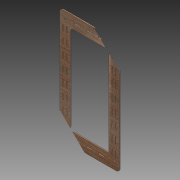
# Autodesk Inventor part: prim
Saved by Autodesk Inventor 2015 (Build 190159000, 159)
## iProperties
Created: 2015-12-31
Part Number: prim
Material: Generic
Document SubType Name: Modeling
Designer: david
Density: 1 g/cm^3
Appearance: Birch - Natural Polished
Author: david
Autodesk Inventor part; units mm, degrees
ref_plane "YZ Plane" through (0, 0, 0) normal (1, 0, 0) x (0, 1, 0)
ref_plane "XZ Plane" through (0, 0, 0) normal (0, 1, 0) x (-1, 0, 0)
ref_plane "XY Plane" through (0, 0, 0) normal (0, 0, 1) x (1, 0, 0)
sketch "Sketch1" plane through (0, 0, 0) normal (0, 1, 0) x (-1, 0, 0)
  line L0 (-100, 190) -> (100, 190)
  line L1 (100, 190) -> (100, -190)
  line L2 (100, -190) -> (-100, -190)
  line L3 (-100, -190) -> (-100, 190)
  line L4 (-100, 190) -> (100, -190) construction
  line L5 (100, 190) -> (-100, -190) construction
  point P0 (0, 0)
  dimension "d0" = 200
  dimension "d1" = 380
  constraints: 12 end point, 2 midpoint, 2 parallel, 1 horizontal, 1 perpendicular
  measures "d0" distance of L1.end L2.end
  measures "d1" distance of L0.end L1.end
extrude "Extrusion1" add sketch "Sketch1" along normal blind 3
sketch "Sketch2" plane through (0, 3, 0) normal (0, 1, 0) x (1, 0, 0)
  line L0 (65, 150) -> (-65, 150)
  line L1 (-65, 150) -> (-65, -150)
  line L2 (-65, -150) -> (65, -150)
  line L3 (65, -150) -> (65, 150)
  line L4 (65, 150) -> (-65, -150) construction
  line L5 (-65, 150) -> (65, -150) construction
  point P0 (0, 0)
  dimension "d4" = 130
  dimension "d5" = 300
  constraints: 12 end point, 2 midpoint, 2 parallel, 1 horizontal, 1 perpendicular
  measures "d4" distance of L2.end L1.end
  measures "d5" distance of L1.end L0.end
extrude "Extrusion2" cut sketch "Sketch2" against normal blind 4
sketch "Sketch3" plane through (0, 3, 0) normal (0, 1, 0) x (1, 0, 0)
  line L0 (100, 190) -> (100, -190) projected
  line L1 (-100, 190) -> (-100, -190) projected
  line L2 (-30.7, 170.55) -> (-51, 170.55)
  line L3 (-51, 170.55) -> (-51, 167.25)
  line L4 (-51, 167.25) -> (-30.7, 167.25)
  line L5 (-30.7, 167.25) -> (-30.7, 170.55)
  line L6 (-30.7, 170.55) -> (-51, 167.25) construction
  line L7 (-51, 170.55) -> (-30.7, 167.25) construction
  line L8 (100, 190) -> (-100, 190) projected
  line L9 (-50.3, -168.2) -> (-30, -168.2)
  line L10 (-30, -168.2) -> (-30, -171.5)
  line L11 (-30, -171.5) -> (-50.3, -171.5)
  line L12 (-50.3, -171.5) -> (-50.3, -168.2)
  line L13 (-50.3, -168.2) -> (-30, -171.5) construction
  line L14 (-30, -168.2) -> (-50.3, -171.5) construction
  line L15 (-100, -190) -> (100, -190) projected
  point P0 (0, 0)
  point P1 (-40.85, 168.9)
  point P2 (-40.15, -169.85)
  dimension "d21" = 20.3
  dimension "d22" = 3.3
  dimension "d24" = 20.3
  dimension "d25" = 3.3
  dimension "d26" = 18.5
  dimension "d32" = 49.7
  dimension "d33" = 49
  dimension "d34" = 22.75
  constraints: 24 end point, 4 midpoint, 4 parallel, 2 horizontal, 2 perpendicular
  measures "d21" distance of L4.end L3.end
  measures "d22" distance of L3.end L2.end
  measures "d24" distance of L10.end L11.end
  measures "d25" distance of L9.end L10.end
  measures "d26" distance between parallel lines of L15 L11
  measures "d32" distance between parallel lines of L1 L12
  measures "d33" distance between parallel lines of L1 L3
  measures "d34" distance between parallel lines of L8 L4
extrude "Extrusion3" cut sketch "Sketch3" against normal blind 4 contours L5 L4 L3 L2 | L9 L10 L11 L12
sketch "Sketch4" plane through (0, 0, 0) normal (0, -1, 0) x (1, 0, 0)
  line L0 (-87.2, 127.35) -> (-90.5, 127.35)
  line L1 (-90.5, 127.35) -> (-90.5, 147.65)
  line L2 (-90.5, 147.65) -> (-87.2, 147.65)
  line L3 (-87.2, 147.65) -> (-87.2, 127.35)
  line L4 (-87.2, 127.35) -> (-90.5, 147.65) construction
  line L5 (-90.5, 127.35) -> (-87.2, 147.65) construction
  line L6 (100, 190) -> (-100, 190) projected
  line L7 (-100, 190) -> (-100, -190) projected
  line L8 (-75.35, 147.65) -> (-78.65, 147.65)
  line L9 (-78.65, 147.65) -> (-78.65, 127.35)
  line L10 (-78.65, 127.35) -> (-75.35, 127.35)
  line L11 (-75.35, 127.35) -> (-75.35, 147.65)
  line L12 (-75.35, 147.65) -> (-78.65, 127.35) construction
  line L13 (-78.65, 147.65) -> (-75.35, 127.35) construction
  line L14 (85.65, 127.35) -> (88.95, 127.35)
  line L15 (88.95, 127.35) -> (88.95, 147.65)
  line L16 (88.95, 147.65) -> (85.65, 147.65)
  line L17 (85.65, 147.65) -> (85.65, 127.35)
  line L18 (85.65, 127.35) -> (88.95, 147.65) construction
  line L19 (88.95, 127.35) -> (85.65, 147.65) construction
  line L20 (75.35, 147.65) -> (78.65, 147.65)
  line L21 (78.65, 147.65) -> (78.65, 127.35)
  line L22 (78.65, 127.35) -> (75.35, 127.35)
  line L23 (75.35, 127.35) -> (75.35, 147.65)
  line L24 (75.35, 147.65) -> (78.65, 127.35) construction
  line L25 (78.65, 147.65) -> (75.35, 127.35) construction
  line L26 (65, 150) -> (65, -150) projected
  line L27 (-65, 150) -> (65, 150) projected
  point P0 (0, 0)
  point P1 (-88.85, 137.5)
  point P2 (-77, 137.5)
  point P3 (87.3, 137.5)
  point P4 (77, 137.5)
  dimension "d35" = 3.3
  dimension "d36" = 20.3
  dimension "d37" = 42.35
  dimension "d38" = 9.5
  dimension "d39" = 3.3
  dimension "d40" = 20.3
  dimension "d41" = 8.55
  dimension "d47" = 42.35
  dimension "d80" = 20.3
  dimension "d81" = 10.35
  dimension "d82" = 7
  dimension "d83" = 2.35
  dimension "d84" = 2.35
  dimension "d85" = 3.3
  dimension "d86" = 3.3
  constraints: 48 end point, 8 midpoint, 4 parallel, 2 horizontal, 2 perpendicular
  measures "d35" distance of L1.end L2.end
  measures "d36" distance of L0.end L1.end
  measures "d37" distance between parallel lines of L2 L6
  measures "d38" distance between parallel lines of L7 L1
  measures "d39" distance of L10.end L9.end
  measures "d40" distance of L9.end L8.end
  measures "d41" distance between parallel lines of L3 L9
  measures "d47" distance between parallel lines of L8 L6
  measures "d80" distance of L22.end L20.start
  measures "d81" distance between parallel lines of L26 L23
  measures "d82" distance between parallel lines of L17 L21
  measures "d83" distance between parallel lines of L27 L16
  measures "d84" distance between parallel lines of L27 L20
  measures "d85" distance of L21.end L22.end
  measures "d86" distance of L14.start L14.end
extrude "Extrusion4" cut sketch "Sketch4" against normal blind 10
pattern_linear "Rectangular Pattern1" count 8 spacing 40 along (0, 0, -1) of "Extrusion4"
sketch "Sketch5" plane through (0, 0, 0) normal (0, -1, 0) x (1, 0, 0)
  circle A0 centre (-82.5, 165) radius 3.5
  circle A1 centre (-82.5, -163) radius 3.5
  circle A2 centre (82.5, -163) radius 3.5
  circle A3 centre (82.5, 165) radius 3.5
  line L0 (85.65, 147.65) -> (88.95, 147.65) projected
  line L1 (100, -190) -> (100, 190) projected
  line L2 (88.95, -152.65) -> (85.65, -152.65) projected
  line L3 (-75.35, -152.65) -> (-78.65, -152.65) projected
  line L4 (-65, -150) -> (-65, 150) projected
  line L5 (-90.5, 147.65) -> (-87.2, 147.65) projected
  circle A4 centre (-82.5, -2.5) radius 3.5
  circle A5 centre (86.5, -2.5) radius 3.5
  line L6 (100, 190) -> (-100, 190) projected
  line L7 (-100, -190) -> (100, -190) projected
  line L8 (-100, 190) -> (-100, -190) projected
  point P0 (0, 0)
  dimension "d48" = 7
  dimension "d49" = 7
  dimension "d50" = 7
  dimension "d51" = 7
  dimension "d53" = 17.5
  dimension "d54" = 17.5
  dimension "d65" = 7
  dimension "d66" = 160.5
  dimension "d67" = 167.5
  dimension "d68" = 7
  dimension "d69" = 167.5
  dimension "d70" = 160.5
  dimension "d71" = 25
  dimension "d72" = 27
  dimension "d73" = 27
  dimension "d76" = 17.5
  dimension "d77" = 17.5
  dimension "d78" = 25
  constraints: 6 centre point
  measures "d48" diameter of A0
  measures "d49" diameter of A1
  measures "d50" diameter of A2
  measures "d51" diameter of A3
  measures "d53" distance from line of L1 A3.centre
  measures "d54" distance from line of L1 A2.centre
  measures "d65" diameter of A4
  measures "d66" distance of A1.centre A4.centre
  measures "d67" distance of A0.centre A4.centre
  measures "d68" diameter of A5
  measures "d69" vertical distance of A5.centre A3.centre
  measures "d70" vertical distance of A2.centre A5.centre
  measures "d71" distance from line of A3.centre L6
  measures "d72" distance from line of L7 A2.centre
  measures "d73" distance from line of L7 A1.centre
  measures "d76" distance from line of L8 A4.centre
  measures "d77" distance from line of L4 A0.centre
  measures "d78" distance from line of L6 A0.centre
extrude "Extrusion5" cut sketch "Sketch5" against normal blind 10 contours A0 | A1 | A2 | A3
pattern_linear "Rectangular Pattern2" count 3 spacing 40 along (1, 0, 0) of "Extrusion3"
fillet "Fillet1" radius 10 6 edges at (-100, 1.5, -190) (100, 1.5, -190) (100, 1.5, 190) (-100, 1.5, 190) (-65, 1.5, -150) (-65, 1.5, 150)
body "Solid1"
